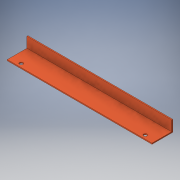
# Autodesk Inventor part: CU2
Saved by Autodesk Inventor 2016 (Build 200138000, 138)
## iProperties
Created: 2018-04-30
Part Number: CU2
Material: Copper
Document SubType Name: Modeling
Designer: Phil Erle
Density: 8.94 g/cm^3
Appearance: Copper - Satin
Author: Phil Erle
Autodesk Inventor part; units mm, degrees
ref_plane "YZ Plane" through (0, 0, 0) normal (1, 0, 0) x (0, 1, 0)
ref_plane "XZ Plane" through (0, 0, 0) normal (0, 1, 0) x (-1, 0, 0)
ref_plane "XY Plane" through (0, 0, 0) normal (0, 0, 1) x (1, 0, 0)
sketch "Sketch1" plane through (0, 0, 0) normal (0, 0, 1) x (1, 0, 0)
  line L0 (-70, -10) -> (70, -10)
  line L1 (70, -10) -> (70, 10)
  line L2 (70, 10) -> (-70, 10)
  line L3 (-70, 10) -> (-70, -10)
  line L4 (-70, -10) -> (70, 10) construction
  line L5 (70, -10) -> (-70, 10) construction
  point P0 (0, 0)
  dimension "d0" = 140
  dimension "d1" = 20
  constraints: 12 end point, 2 midpoint, 2 parallel, 1 horizontal, 1 perpendicular
  measures "d0" distance of L2.end L1.end
  measures "d1" distance of L2.end L0.start
extrude "Extrusion1" add sketch "Sketch1" along normal blind 1
sketch "Sketch2" plane through (0, 0, 1) normal (0, 0, 1) x (1, 0, 0)
  line L0 (70, 10) -> (-70, 10) projected
  line L1 (-70, 10) -> (70, 10)
  line L2 (70, 10) -> (70, 9)
  line L3 (70, 9) -> (-70, 9)
  line L4 (-70, 9) -> (-70, 10)
  point P0 (0, 0)
  dimension "d4" = 1
  constraints: 8 end point, 2 parallel, 1 horizontal, 1 perpendicular
  measures "d4" distance of L1.end L2.end
extrude "Extrusion2" add sketch "Sketch2" along normal blind 10
sketch "Sketch3" plane through (0, 0, 1) normal (0, 0, 1) x (1, 0, 0)
  line L0 (-60, -6.5) -> (60, -6.5) construction
  line L1 (-70, -10) -> (70, -10) construction
  point P0 (0, 0)
  point P1 (0, -6.5)
  dimension "d7" = 120
  dimension "d8" = 3.5
  constraints: 2 coincident, 2 end point, 1 horizontal, 1 midpoint, 1 vertical alignment
  measures "d7" distance of L0.start L0.end
  measures "d8" distance between parallel lines of L1 L0
hole "Hole1" at (-60, -6.5, 1) at (60, -6.5, 1) direction (0, 0, -1) diameter 3.4 depth 8 tip angle 118 clearance for "Countersunk Flat Head Screw DIN EN ISO 2009" size "M3" standard "DIN"
body "Solid1"
